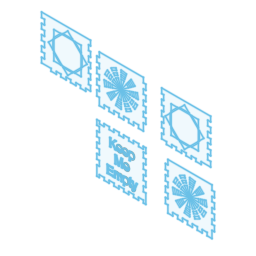
candelholder (Autodesk Fusion 360 design; units mm, degrees)
Autodesk Fusion 360 part; units mm, degrees
(part 1 of 3)
sketch "Sketch1" plane through (0, 0, 0) normal (0, 1, 0) x (1, 0, 0)
  line L0 (0, 0) -> (50, 0)
  line L1 (50, 0) -> (50, -50)
  line L2 (50, -50) -> (0, -50)
  line L3 (0, -50) -> (0, 0)
  line L4 (2.5, 0) -> (2.5, -2.5)
  line L5 (2.5, -2.5) -> (7.5, -2.5)
  line L6 (7.5, -2.5) -> (7.5, 0)
  line L7 (17.5, -2.5) -> (17.5, 0)
  line L8 (12.5, -2.5) -> (17.5, -2.5)
  line L9 (12.5, 0) -> (12.5, -2.5)
  line L10 (27.5, -2.5) -> (27.5, 0)
  line L11 (22.5, -2.5) -> (27.5, -2.5)
  line L12 (22.5, 0) -> (22.5, -2.5)
  line L13 (37.5, -2.5) -> (37.5, 0)
  line L14 (32.5, -2.5) -> (37.5, -2.5)
  line L15 (32.5, 0) -> (32.5, -2.5)
  line L16 (47.5, -2.5) -> (47.5, 0)
  line L17 (42.5, -2.5) -> (47.5, -2.5)
  line L18 (42.5, 0) -> (42.5, -2.5)
  line L19 (50, -25) -> (0, -25) construction
  line L20 (2.5, -50) -> (2.5, -47.5)
  line L21 (7.5, -47.5) -> (7.5, -50)
  line L22 (2.5, -47.5) -> (7.5, -47.5)
  line L23 (12.5, -50) -> (12.5, -47.5)
  line L24 (12.5, -47.5) -> (17.5, -47.5)
  line L25 (17.5, -47.5) -> (17.5, -50)
  line L26 (22.5, -50) -> (22.5, -47.5)
  line L27 (22.5, -47.5) -> (27.5, -47.5)
  line L28 (27.5, -47.5) -> (27.5, -50)
  line L29 (32.5, -50) -> (32.5, -47.5)
  line L30 (32.5, -47.5) -> (37.5, -47.5)
  line L31 (37.5, -47.5) -> (37.5, -50)
  line L32 (42.5, -50) -> (42.5, -47.5)
  line L33 (47.5, -47.5) -> (47.5, -50)
  line L34 (42.5, -47.5) -> (47.5, -47.5)
  line L35 (0, -5) -> (2.5, -5)
  line L36 (2.5, -5) -> (2.5, -10)
  line L37 (2.5, -10) -> (0, -10)
  line L38 (0, -15) -> (2.5, -15)
  line L39 (2.5, -15) -> (2.5, -20)
  line L40 (2.5, -20) -> (0, -20)
  line L41 (0, -25) -> (2.5, -25)
  line L42 (2.5, -25) -> (2.5, -30)
  line L43 (2.5, -30) -> (0, -30)
  line L44 (0, -35) -> (2.5, -35)
  line L45 (2.5, -35) -> (2.5, -40)
  line L46 (2.5, -40) -> (0, -40)
  line L47 (25, 0) -> (25, -50) construction
  line L48 (50, -5) -> (47.5, -5)
  line L49 (47.5, -10) -> (50, -10)
  line L50 (47.5, -5) -> (47.5, -10)
  line L51 (50, -15) -> (47.5, -15)
  line L52 (47.5, -15) -> (47.5, -20)
  line L53 (47.5, -20) -> (50, -20)
  line L54 (47.5, -25) -> (47.5, -30)
  line L55 (47.5, -30) -> (50, -30)
  line L56 (50, -25) -> (47.5, -25)
  line L57 (50, -35) -> (47.5, -35)
  line L58 (47.5, -35) -> (47.5, -40)
  line L59 (47.5, -40) -> (50, -40)
  dimension "d5" = 50
  dimension "d6" = 50
  dimension "d9" = 2.5
  dimension "d10" = 5
  dimension "d14" = 10
  dimension "d15" = 0
  dimension "d19" = 2.5
  dimension "d20" = 5
  dimension "d21" = 5
  dimension "d24" = -10
  dimension "d25" = 0
  constraint horizontal L0
  constraint vertical L1
  constraint horizontal L2
  constraint vertical L3
  constraint coincident L0.start L3.end
  constraint coincident L0 L4.start
  constraint perpendicular L0 L4
  constraint perpendicular L3 L5
  constraint coincident L0 L6.end
  constraint perpendicular L0 L6
  constraint midpoint L1 L19.start
  constraint midpoint L3 L19.end
  constraint symmetric L4.start L19 L20.start
  constraint symmetric L4.end L19 L20.end
  constraint symmetric L5.end L19 L21.start
  constraint symmetric L6.end L19 L21.end
  constraint symmetric L7.start L19 L24.end
  constraint symmetric L7.end L19 L25.end
  constraint symmetric L8.start L19 L23.end
  constraint symmetric L9.start L19 L23.start
  constraint symmetric L10.start L19 L27.end
  constraint symmetric L10.end L19 L28.end
  constraint symmetric L11.start L19 L26.end
  constraint symmetric L12.start L19 L26.start
  constraint symmetric L13.start L19 L30.end
  constraint symmetric L13.end L19 L31.end
  constraint symmetric L14.start L19 L29.end
  constraint symmetric L15.start L19 L29.start
  constraint symmetric L16.start L19 L33.start
  constraint symmetric L16.end L19 L33.end
  constraint symmetric L17.start L19 L32.end
  constraint symmetric L18.start L19 L32.start
  constraint coincident L3 L35.start
  constraint perpendicular L3 L35
  constraint perpendicular L19 L36
  constraint coincident L3 L37.end
  constraint perpendicular L3 L37
  constraint midpoint L0 L47.start
  constraint midpoint L2 L47.end
  constraint symmetric L35.start L47 L48.start
  constraint symmetric L35.end L47 L48.end
  constraint symmetric L36.end L47 L49.start
  constraint symmetric L37.end L47 L49.end
  constraint symmetric L38.start L47 L51.start
  constraint symmetric L38.end L47 L51.end
  constraint symmetric L39.end L47 L52.end
  constraint symmetric L40.end L47 L53.end
  constraint symmetric L19.end L47 L19.start
  constraint symmetric L41.end L47 L54.start
  constraint symmetric L42.end L47 L54.end
  constraint symmetric L43.end L47 L55.end
  constraint symmetric L44.start L47 L57.start
  constraint symmetric L44.end L47 L57.end
  constraint symmetric L45.end L47 L58.end
  constraint symmetric L46.end L47 L59.end
  measures "d5" distance of L0.start L0.end
  measures "d6" distance of L0.start L2.end
  measures "d9" distance of L4.start L4.end
  measures "d10" distance of L4.end L5.end
  measures "d19" distance of L35.start L35.end
  measures "d20" distance of L35.end L36.end
  measures "d21" distance of L0.start L35
extrude "Extrude1" add sketch "Sketch1" along normal blind 3 contours L0 L1 L2 L3 L4 L5 L6 L7 L8 L9 L10 L11 L12 L13 L14 L15 L16 L17 L18 L20 L21 L22 L23 L24 L25 L26 L27 L28 L29 L30 L31 L32 L33 L34 L35 L36 L37 L38 L39 L40 L41 L42 L43 L44 L45 L46 L48 L49 L50 L51 L52 L53 L54 L55 L56 L57 L58 L59 makes body 1
sketch "Sketch2" plane through (0, 0, 0) normal (1, 0, 0) x (0, 0, -1)
  line L0 (-46.9428, 61.6884) -> (3.0572, 61.6884)
  line L1 (3.0572, 61.6884) -> (3.0572, 11.6884)
  line L2 (3.0572, 11.6884) -> (-46.9428, 11.6884)
  line L3 (-46.9428, 11.6884) -> (-46.9428, 61.6884)
  line L4 (-7.7428, 61.6884) -> (-7.7428, 59.1884)
  line L5 (-7.7428, 59.1884) -> (-2.3428, 59.1884)
  line L6 (-2.3428, 59.1884) -> (-2.3428, 61.6884)
  line L7 (-12.3428, 59.1884) -> (-12.3428, 61.6884)
  line L8 (-17.7428, 59.1884) -> (-12.3428, 59.1884)
  line L9 (-17.7428, 61.6884) -> (-17.7428, 59.1884)
  line L10 (-22.3428, 59.1884) -> (-22.3428, 61.6884)
  line L11 (-27.7428, 59.1884) -> (-22.3428, 59.1884)
  line L12 (-27.7428, 61.6884) -> (-27.7428, 59.1884)
  line L13 (-32.3428, 59.1884) -> (-32.3428, 61.6884)
  line L14 (-37.7428, 59.1884) -> (-32.3428, 59.1884)
  line L15 (-37.7428, 61.6884) -> (-37.7428, 59.1884)
  line L16 (3.0572, 36.6884) -> (-46.9428, 36.6884) construction
  line L17 (-21.9428, 61.6884) -> (-21.9428, 11.6884) construction
  line L18 (-37.7428, 11.6884) -> (-37.7428, 14.1884)
  line L19 (-32.3428, 14.1884) -> (-32.3428, 11.6884)
  line L20 (-27.7428, 11.6884) -> (-27.7428, 14.1884)
  line L21 (-22.3428, 14.1884) -> (-22.3428, 11.6884)
  line L22 (-17.7428, 11.6884) -> (-17.7428, 14.1884)
  line L23 (-12.3428, 14.1884) -> (-12.3428, 11.6884)
  line L24 (-7.7428, 11.6884) -> (-7.7428, 14.1884)
  line L25 (-2.3428, 14.1884) -> (-2.3428, 11.6884)
  line L26 (3.0572, 59.1884) -> (0.5572, 59.1884)
  line L27 (0.5572, 54.1884) -> (3.0572, 54.1884)
  line L28 (3.0572, 49.1884) -> (0.5572, 49.1884)
  line L29 (0.5572, 44.1884) -> (3.0572, 44.1884)
  line L30 (3.0572, 39.1884) -> (0.5572, 39.1884)
  line L31 (0.5572, 36.6884) -> (0.5572, 34.1884)
  line L32 (0.5572, 34.1884) -> (3.0572, 34.1884)
  line L33 (3.0572, 29.1884) -> (0.5572, 29.1884)
  line L34 (0.5572, 24.1884) -> (3.0572, 24.1884)
  line L35 (3.0572, 19.1884) -> (0.5572, 19.1884)
  line L36 (0.5572, 14.1884) -> (3.0572, 14.1884)
  line L37 (-46.9428, 59.1884) -> (-44.4428, 59.1884)
  line L38 (-44.4428, 54.1884) -> (-46.9428, 54.1884)
  line L39 (-44.4428, 44.1884) -> (-46.9428, 44.1884)
  line L40 (-46.9428, 49.1884) -> (-44.4428, 49.1884)
  line L41 (-46.9428, 39.1884) -> (-44.4428, 39.1884)
  line L42 (-44.4428, 34.1884) -> (-46.9428, 34.1884)
  line L43 (-46.9428, 29.1884) -> (-44.4428, 29.1884)
  line L44 (-44.4428, 24.1884) -> (-46.9428, 24.1884)
  line L45 (-46.9428, 19.1884) -> (-44.4428, 19.1884)
  line L46 (-44.4428, 14.1884) -> (-46.9428, 14.1884)
  line L47 (-44.4428, 59.1884) -> (-37.7428, 59.1884)
  line L48 (-44.4428, 14.1884) -> (-37.7428, 14.1884)
  line L49 (0.5572, 14.1884) -> (-2.3428, 14.1884)
  line L50 (-2.3428, 59.1884) -> (0.5572, 59.1884)
  line L51 (-7.7428, 59.1884) -> (-32.3428, 59.1884)
  line L52 (0.5572, 49.1884) -> (0.5572, 54.1884)
  line L53 (-44.4428, 24.1884) -> (-44.4428, 19.1884)
  line L54 (-44.4428, 34.1884) -> (-44.4428, 29.1884)
  line L55 (-44.4428, 54.1884) -> (-44.4428, 49.1884)
  line L56 (-44.4428, 44.1884) -> (-44.4428, 39.1884)
  line L57 (-27.7428, 14.1884) -> (-32.3428, 14.1884)
  line L58 (-7.7428, 14.1884) -> (-12.3428, 14.1884)
  line L59 (-17.7428, 14.1884) -> (-22.3428, 14.1884)
  line L60 (0.5572, 19.1884) -> (0.5572, 24.1884)
  line L61 (0.5572, 29.1884) -> (0.5572, 36.6884)
  line L62 (0.5572, 39.1884) -> (0.5572, 44.1884)
  dimension "d29" = 50
  dimension "d30" = 50
  dimension "d31" = 2.5
  dimension "d32" = 5.4
  dimension "d33" = 5.4
  dimension "d36" = -10
  dimension "d37" = 0
  dimension "d38" = 2.5
  dimension "d39" = 5
  dimension "d40" = 2.5
  constraint horizontal L0
  constraint vertical L1
  constraint horizontal L2
  constraint vertical L3
  constraint coincident L0 L4.start
  constraint perpendicular L0 L4
  constraint perpendicular L4 L5
  constraint coincident L0 L6.end
  constraint perpendicular L0 L6
  constraint midpoint L1 L16.start
  constraint midpoint L3 L16.end
  constraint midpoint L0 L17.start
  constraint midpoint L2 L17.end
  constraint symmetric L4.start L16 L24.start
  constraint symmetric L4.end L16 L24.end
  constraint symmetric L5.end L16 L25.start
  constraint symmetric L6.end L16 L25.end
  constraint symmetric L7.start L16 L23.start
  constraint symmetric L7.end L16 L23.end
  constraint symmetric L8.start L16 L22.end
  constraint symmetric L9.start L16 L22.start
  constraint symmetric L10.start L16 L21.start
  constraint symmetric L10.end L16 L21.end
  constraint symmetric L11.start L16 L20.end
  constraint symmetric L12.start L16 L20.start
  constraint symmetric L13.start L16 L19.start
  constraint symmetric L13.end L16 L19.end
  constraint symmetric L14.start L16 L18.end
  constraint symmetric L15.start L16 L18.start
  constraint coincident L1 L26.start
  constraint perpendicular L1 L26
  constraint coincident L1 L27.end
  constraint perpendicular L1 L27
  constraint symmetric L17 L26.start L37.start
  constraint symmetric L17 L26.end L37.end
  constraint symmetric L17 L27.start L38.start
  constraint symmetric L17 L27.end L38.end
  constraint symmetric L17 L28.start L40.start
  constraint symmetric L17 L28.end L40.end
  constraint symmetric L17 L29.start L39.start
  constraint symmetric L17 L29.end L39.end
  constraint symmetric L17 L30.start L41.start
  constraint symmetric L17 L30.end L41.end
  constraint symmetric L17 L31.end L42.start
  constraint symmetric L17 L32.end L42.end
  constraint symmetric L17 L33.start L43.start
  constraint symmetric L17 L33.end L43.end
  constraint symmetric L17 L34.start L44.start
  constraint symmetric L17 L34.end L44.end
  constraint symmetric L17 L35.start L45.start
  constraint symmetric L17 L35.end L45.end
  constraint symmetric L17 L36.start L46.start
  constraint symmetric L17 L36.end L46.end
  constraint collinear L53 L55
  constraint collinear L54 L55
  constraint collinear L55 L56
  constraint collinear L57 L58
  constraint collinear L58 L59
  constraint collinear L60 L61
  constraint coincident L16 L31.start
  constraint collinear L61 L62
  measures "d29" distance of L0.start L0.end
  measures "d30" distance of L0.start L2.end
  measures "d31" distance of L4.start L4.end
  measures "d32" distance of L4.end L5.end
  measures "d33" horizontal distance of L0.end L5.end
  measures "d38" distance of L26.start L26.end
  measures "d39" distance of L26.end L27.start
  measures "d40" distance of L0 L26
extrude "Extrude2" add sketch "Sketch2" along normal blind 3 separate body contours L1 L2 L3 L5 L8 L11 L14 L18 L19 L20 L21 L22 L23 L24 L25 L26 L27 L28 L29 L30 L32 L33 L34 L35 L36 L37 L38 L39 L40 L41 L42 L43 L44 L45 L46 L47 L48 L49 L50 L51 L52 L53 L54 L55 L56 L57 L58 L59 L60 L61 L62 makes body 2
copy_body "Body->Comp1" bodies 1 removing the originals makes body 3 in component "Component"
copy_body "Body->Comp3" bodies 2 removing the originals makes body 4 in component "Component''"
extrude "Extrude1'" cut 5 faces at (1, 27.5218, -3.0572) (1, 17.5218, -3.0572) (1, 37.5218, -3.0572) (1, 47.5218, -3.0572) (1, 57.5218, -3.0572) along direction (0, 0, 1) blind 0.5 on bodies 4 bodies 4 in component "Component''"
extrude "Extrude2'" add 5 faces at (1, 25.8551, 46.9428) (1, 15.8551, 46.9428) (1, 35.8551, 46.9428) (1, 45.8551, 46.9428) (1, 55.8551, 46.9428) along direction (0, 0, 1) blind 0.5 on bodies 4 bodies 4 in component "Component''"
sketch "Sketch3" plane through (0, 0, 0) normal (0, 0, 1) x (1, 0, 0)
  line L0 (0, 0) -> (50, 0)
  line L1 (50, 0) -> (50, 47.5)
  line L2 (50, 47.5) -> (0, 47.5)
  line L3 (0, 47.5) -> (0, 0)
  line L4 (47.5, 37.5) -> (47.5, 42.5)
  line L5 (47.5, 42.5) -> (50.5, 42.5)
  line L6 (50.5, 42.5) -> (50.5, 37.5)
  line L7 (50.5, 37.5) -> (47.5, 37.5)
  line L8 (47.5, 27.5) -> (47.5, 32.5)
  line L9 (47.5, 32.5) -> (50.5, 32.5)
  line L10 (50.5, 32.5) -> (50.5, 27.5)
  line L11 (50.5, 27.5) -> (47.5, 27.5)
  line L12 (47.5, 17.5) -> (47.5, 22.5)
  line L13 (47.5, 22.5) -> (50.5, 22.5)
  line L14 (50.5, 22.5) -> (50.5, 17.5)
  line L15 (50.5, 17.5) -> (47.5, 17.5)
  line L16 (47.5, 7.5) -> (47.5, 12.5)
  line L17 (47.5, 12.5) -> (50.5, 12.5)
  line L18 (50.5, 12.5) -> (50.5, 7.5)
  line L19 (50.5, 7.5) -> (47.5, 7.5)
  line L20 (47.5, 0) -> (42.5, 0)
  line L21 (42.5, 0) -> (42.5, 3)
  line L22 (42.5, 3) -> (47.5, 3)
  line L23 (47.5, 3) -> (47.5, 0)
  line L24 (37.5, 0) -> (32.5, 0)
  line L25 (32.5, 0) -> (32.5, 3)
  line L26 (32.5, 3) -> (37.5, 3)
  line L27 (37.5, 3) -> (37.5, 0)
  line L28 (27.5, 0) -> (22.5, 0)
  line L29 (22.5, 0) -> (22.5, 3)
  line L30 (22.5, 3) -> (27.5, 3)
  line L31 (27.5, 3) -> (27.5, 0)
  line L32 (17.5, 0) -> (12.5, 0)
  line L33 (12.5, 0) -> (12.5, 3)
  line L34 (12.5, 3) -> (17.5, 3)
  line L35 (17.5, 3) -> (17.5, 0)
  line L36 (7.5, 0) -> (2.5, 0)
  line L37 (2.5, 0) -> (2.5, 3)
  line L38 (2.5, 3) -> (7.5, 3)
  line L39 (7.5, 3) -> (7.5, 0)
  line L40 (-0.5, 7.5) -> (-0.5, 12.5)
  line L41 (-0.5, 12.5) -> (2.5, 12.5)
  line L42 (2.5, 12.5) -> (2.5, 7.5)
  line L43 (2.5, 7.5) -> (-0.5, 7.5)
  line L44 (-0.5, 17.5) -> (-0.5, 22.5)
  line L45 (-0.5, 22.5) -> (2.5, 22.5)
  line L46 (2.5, 22.5) -> (2.5, 17.5)
  line L47 (2.5, 17.5) -> (-0.5, 17.5)
  line L48 (-0.5, 27.5) -> (-0.5, 32.5)
  line L49 (-0.5, 32.5) -> (2.5, 32.5)
  line L50 (2.5, 32.5) -> (2.5, 27.5)
  line L51 (2.5, 27.5) -> (-0.5, 27.5)
  line L52 (-0.5, 37.5) -> (-0.5, 42.5)
  line L53 (-0.5, 42.5) -> (2.5, 42.5)
  line L54 (2.5, 42.5) -> (2.5, 37.5)
  line L55 (2.5, 37.5) -> (-0.5, 37.5)
  line L56 (2.5, 42.5) -> (2.5, 47.5)
  line L57 (2.5, 32.5) -> (2.5, 37.5)
  line L58 (2.5, 22.5) -> (2.5, 27.5)
  line L59 (2.5, 12.5) -> (2.5, 17.5)
  line L60 (2.5, 2.5) -> (2.5, 7.5)
  line L61 (47.5, 42.5) -> (50.5, 42.5)
  line L62 (50.5, 32.5) -> (50.5, 37.5)
  line L63 (50.5, 37.5) -> (50.5, 42.5)
  line L64 (50.5, 42.5) -> (50.5, 47.5)
  line L65 (50.5, 47.5) -> (50.5, 42.5)
  line L66 (50.5, 42.5) -> (50.5, 37.5)
  line L67 (50.5, 37.5) -> (50.5, 32.5)
  line L68 (50.5, 32.5) -> (50.5, 27.5)
  line L69 (50.5, 27.5) -> (50.5, 22.5)
  line L70 (50.5, 22.5) -> (50.5, 17.5)
  line L71 (50.5, 17.5) -> (50.5, 12.5)
  line L72 (50.5, 12.5) -> (50.5, 7.5)
  line L73 (50.5, 7.5) -> (50.5, 2.5)
  line L74 (50.5, 2.5) -> (50.5, 0)
  line L75 (50.5, 0) -> (50.5, 2.5)
  line L76 (50.5, 2.5) -> (50.5, 0)
  line L77 (50.5, 0) -> (50.5, 2.5)
  line L78 (50.5, 2.5) -> (50.5, 0)
  line L79 (50.5, 0) -> (50.5, 2.5)
  line L80 (50.5, 2.5) -> (50.5, 0)
  line L81 (50.5, 0) -> (50.5, 2.5)
  line L82 (50.5, 2.5) -> (50.5, 7.5)
  line L83 (50.5, 7.5) -> (50.5, 12.5)
  line L84 (50.5, 12.5) -> (50.5, 17.5)
  line L85 (50.5, 17.5) -> (50.5, 22.5)
  line L86 (50.5, 22.5) -> (50.5, 27.5)
  line L87 (50.5, 27.5) -> (50.5, 32.5)
  line L88 (-0.5, 37.5) -> (-0.5, 32.5)
  line L89 (-0.5, 32.5) -> (-0.5, 27.5)
  line L90 (-0.5, 27.5) -> (-0.5, 22.5)
  line L91 (-0.5, 22.5) -> (-0.5, 17.5)
  line L92 (-0.5, 17.5) -> (-0.5, 12.5)
  line L93 (-0.5, 12.5) -> (-0.5, 7.5)
  line L94 (-0.5, 7.5) -> (-0.5, 2.5)
  line L95 (-0.5, 2.5) -> (-0.5, 0)
  line L96 (-0.5, 0) -> (-0.5, 2.5)
  line L97 (-0.5, 2.5) -> (-0.5, 0)
  line L98 (-0.5, 0) -> (-0.5, 2.5)
  line L99 (-0.5, 2.5) -> (-0.5, 0)
  line L100 (-0.5, 0) -> (-0.5, 2.5)
  line L101 (-0.5, 2.5) -> (-0.5, 0)
  line L102 (-0.5, 0) -> (-0.5, 2.5)
  line L103 (-0.5, 2.5) -> (-0.5, 7.5)
  line L104 (-0.5, 7.5) -> (-0.5, 12.5)
  line L105 (-0.5, 12.5) -> (-0.5, 17.5)
  line L106 (-0.5, 17.5) -> (-0.5, 22.5)
  line L107 (-0.5, 22.5) -> (-0.5, 27.5)
  line L108 (-0.5, 27.5) -> (-0.5, 32.5)
  line L109 (-0.5, 32.5) -> (-0.5, 37.5)
  line L110 (-0.5, 37.5) -> (-0.5, 42.5)
  line L111 (-0.5, 42.5) -> (-0.5, 47.5)
  line L112 (-0.5, 47.5) -> (-0.5, 42.5)
  line L113 (-0.5, 42.5) -> (-0.5, 37.5)
  line L114 (2.5, 0) -> (0, 0)
  line L115 (0, 0) -> (2.5, 0)
  line L116 (2.5, 0) -> (7.5, 0)
  line L117 (7.5, 0) -> (12.5, 0)
  line L118 (12.5, 0) -> (17.5, 0)
  line L119 (17.5, 0) -> (22.5, 0)
  line L120 (22.5, 0) -> (27.5, 0)
  line L121 (27.5, 0) -> (32.5, 0)
  line L122 (32.5, 0) -> (37.5, 0)
  line L123 (37.5, 0) -> (42.5, 0)
  line L124 (42.5, 0) -> (47.5, 0)
  line L125 (47.5, 0) -> (50, 0)
  line L126 (50, 0) -> (47.5, 0)
  line L127 (47.5, 0) -> (50, 0)
  line L128 (50, 0) -> (47.5, 0)
  line L129 (47.5, 0) -> (50, 0)
  line L130 (50, 0) -> (47.5, 0)
  line L131 (47.5, 0) -> (50, 0)
  line L132 (50, 0) -> (47.5, 0)
  line L133 (47.5, 0) -> (50, 0)
  line L134 (50, 0) -> (47.5, 0)
  line L135 (47.5, 0) -> (42.5, 0)
  line L136 (42.5, 0) -> (37.5, 0)
  line L137 (37.5, 0) -> (32.5, 0)
  line L138 (32.5, 0) -> (27.5, 0)
  line L139 (27.5, 0) -> (22.5, 0)
  line L140 (22.5, 0) -> (17.5, 0)
  line L141 (17.5, 0) -> (12.5, 0)
  line L142 (12.5, 0) -> (7.5, 0)
  line L143 (7.5, 0) -> (2.5, 0)
  line L144 (2.5, 0) -> (0, 0)
  line L145 (0, 0) -> (2.5, 0)
  line L146 (2.5, 0) -> (0, 0)
  line L147 (0, 0) -> (2.5, 0)
  line L148 (2.5, 0) -> (0, 0)
  line L149 (0, 0) -> (2.5, 0)
  line L150 (2.5, 0) -> (0, 0)
  line L151 (0, 0) -> (2.5, 0)
  line L152 (47.5, 37.5) -> (47.5, 32.5)
  line L153 (47.5, 32.5) -> (47.5, 27.5)
  line L154 (47.5, 27.5) -> (47.5, 22.5)
  line L155 (47.5, 22.5) -> (47.5, 17.5)
  line L156 (47.5, 17.5) -> (47.5, 12.5)
  line L157 (47.5, 12.5) -> (47.5, 7.5)
  line L158 (47.5, 7.5) -> (47.5, 2.5)
  line L159 (47.5, 2.5) -> (47.5, 0)
  line L160 (47.5, 0) -> (47.5, 2.5)
  line L161 (47.5, 2.5) -> (47.5, 0)
  line L162 (47.5, 0) -> (47.5, 2.5)
  line L163 (47.5, 2.5) -> (47.5, 0)
  line L164 (47.5, 0) -> (47.5, 2.5)
  line L165 (47.5, 2.5) -> (47.5, 0)
  line L166 (47.5, 0) -> (47.5, 2.5)
  line L167 (47.5, 2.5) -> (47.5, 7.5)
  line L168 (47.5, 7.5) -> (47.5, 12.5)
  line L169 (47.5, 12.5) -> (47.5, 17.5)
  line L170 (47.5, 17.5) -> (47.5, 22.5)
  line L171 (47.5, 22.5) -> (47.5, 27.5)
  line L172 (47.5, 27.5) -> (47.5, 32.5)
  line L173 (47.5, 32.5) -> (47.5, 37.5)
  line L174 (47.5, 37.5) -> (47.5, 42.5)
  line L175 (47.5, 42.5) -> (47.5, 47.5)
  line L176 (47.5, 47.5) -> (47.5, 42.5)
  line L177 (47.5, 42.5) -> (47.5, 37.5)
  line L178 (0, 3) -> (2.5, 3)
  line L179 (2.5, 3) -> (0, 3)
  line L180 (0, 3) -> (2.5, 3)
  line L181 (2.5, 3) -> (0, 3)
  line L182 (0, 3) -> (2.5, 3)
  line L183 (2.5, 3) -> (0, 3)
  line L184 (0, 3) -> (2.5, 3)
  line L185 (2.5, 3) -> (0, 3)
  line L186 (0, 3) -> (2.5, 3)
  line L187 (2.5, 3) -> (7.5, 3)
  line L188 (7.5, 3) -> (12.5, 3)
  line L189 (12.5, 3) -> (17.5, 3)
  line L190 (17.5, 3) -> (22.5, 3)
  line L191 (22.5, 3) -> (27.5, 3)
  line L192 (27.5, 3) -> (32.5, 3)
  line L193 (32.5, 3) -> (37.5, 3)
  line L194 (37.5, 3) -> (42.5, 3)
  line L195 (42.5, 3) -> (47.5, 3)
  line L196 (47.5, 3) -> (50, 3)
  line L197 (50, 3) -> (47.5, 3)
  line L198 (47.5, 3) -> (50, 3)
  line L199 (50, 3) -> (47.5, 3)
  line L200 (47.5, 3) -> (50, 3)
  line L201 (50, 3) -> (47.5, 3)
  line L202 (47.5, 3) -> (50, 3)
  line L203 (50, 3) -> (47.5, 3)
  line L204 (47.5, 3) -> (50, 3)
  line L205 (50, 3) -> (47.5, 3)
  line L206 (47.5, 3) -> (42.5, 3)
  line L207 (42.5, 3) -> (37.5, 3)
  line L208 (37.5, 3) -> (32.5, 3)
  line L209 (32.5, 3) -> (27.5, 3)
  line L210 (27.5, 3) -> (22.5, 3)
  line L211 (22.5, 3) -> (17.5, 3)
  line L212 (17.5, 3) -> (12.5, 3)
  line L213 (12.5, 3) -> (7.5, 3)
  line L214 (7.5, 3) -> (2.5, 3)
  line L215 (2.5, 3) -> (0, 3)
  dimension "d71" = 47.5
  dimension "d72" = 50
  constraint horizontal L0
  constraint vertical L1
  constraint horizontal L2
  constraint vertical L3
  constraint coincident L0.start L3.end
  measures "d71" distance of L0.start L2.end
  measures "d72" distance of L1.end L2.end
sketch "Sketch4" plane through (25, 25.25, -65) normal (0, 0, 1) x (1, 0, 0)
extrude "Extrude3" add sketch "Sketch3" against normal blind 3 separate body contours L0 L36 L37 L38 L39 L60 L116 L143 L187 L214 | L3 L41 L42 L43 | L2 L4 L8 L12 L16 L22 L26 L30 L34 L38 L42 L46 L50 L54 L56 L57 L58 L59 L60 L152 L153 L154 L155 L156 L157 L158 L167 L168 L169 L170 L171 L172 L173 L174 L175 L176 L177 L187 L188 L189 L190 L191 L192 L193 L194 L195 L206 L207 L208 L209 L210 L211 L212 L213 L214 | L0 L32 L33 L34 L35 L118 L141 L189 L212 | L3 L45 L46 L47 | L0 L28 L29 L30 L31 L120 L139 L191 L210 | L3 L49 L50 L51 | L0 L24 L25 L26 L27 L122 L137 L193 L208 | L3 L53 L54 L55 | L0 L20 L21 L22 L23 L124 L135 L158 L159 L160 L161 L162 L163 L164 L165 L166 L167 L195 L206 | L1 L16 L17 L19 L157 L168 | L1 L4 L5 L7 L61 L174 L177 | L1 L12 L13 L15 L155 L170 | L1 L8 L9 L11 L153 L172 makes body 5
extrude "Extrude4" add 1 faces at (0.8333, 42.5, -1) along direction (0, 1, 0) blind 0.2 on bodies 5 bodies 5
extrude "Extrude5" add 1 faces at (1.6667, 37.5, -1) along direction (0, -1, 0) blind 0.2 on bodies 5 bodies 5
extrude "Extrude6" add 1 faces at (1.6667, 27.5, -1) along direction (0, -1, 0) blind 0.2 on bodies 5 bodies 5
extrude "Extrude7" add 1 faces at (1.6667, 17.5, -1) along direction (0, -1, 0) blind 0.2 on bodies 5 bodies 5
extrude "Extrude8" add 1 faces at (1.6667, 7.5, -1) along direction (0, -1, 0) blind 0.2 on bodies 5 bodies 5
extrude "Extrude9" add 1 faces at (0.8333, 32.5, -1) along direction (0, 1, 0) blind 0.2 on bodies 5 bodies 5
extrude "Extrude10" add 1 faces at (0.8333, 22.5, -1) along direction (0, 1, 0) blind 0.2 on bodies 5 bodies 5
extrude "Extrude11" add 1 faces at (0.8333, 12.5, -1) along direction (0, 1, 0) blind 0.2 on bodies 5 bodies 5
extrude "Extrude1''" add 1 faces at (7.5, 1, 1.6667) along direction (-1, 0, 0) blind 0.2 on bodies 3 bodies 3 in component "Component"
extrude "Extrude2''" add 1 faces at (17.5, 1, 1.6667) along direction (-1, 0, 0) blind 0.2 on bodies 3 bodies 3 in component "Component"
extrude "Extrude3'" add 1 faces at (27.5, 1, 1.6667) along direction (-1, 0, 0) blind 0.2 on bodies 3 bodies 3 in component "Component"
extrude "Extrude4'" add 1 faces at (37.5, 1, 1.6667) along direction (-1, 0, 0) blind 0.2 on bodies 3 bodies 3 in component "Component"
extrude "Extrude5'" add 1 faces at (47.5, 1, 1.6667) along direction (-1, 0, 0) blind 0.2 on bodies 3 bodies 3 in component "Component"
extrude "Extrude6'" add 1 faces at (42.5, 1, 0.8333) along direction (1, 0, 0) blind 0.2 on bodies 3 bodies 3 in component "Component"
extrude "Extrude7'" add 1 faces at (32.5, 1, 0.8333) along direction (1, 0, 0) blind 0.2 on bodies 3 bodies 3 in component "Component"
extrude "Extrude8'" add 1 faces at (22.5, 1, 0.8333) along direction (1, 0, 0) blind 0.2 on bodies 3 bodies 3 in component "Component"
extrude "Extrude9'" add 1 faces at (12.5, 1, 0.8333) along direction (1, 0, 0) blind 0.2 on bodies 3 bodies 3 in component "Component"
extrude "Extrude10'" add 1 faces at (2.5, 1, 0.8333) along direction (1, 0, 0) blind 0.2 on bodies 3 bodies 3 in component "Component"
extrude "Extrude12" add 1 faces at (49.1667, 7.5, -1) along direction (0, -1, 0) blind 0.2 on bodies 5 bodies 5
extrude "Extrude13" add 1 faces at (49.1667, 17.5, -1) along direction (0, -1, 0) blind 0.2 on bodies 5 bodies 5
extrude "Extrude14" add 1 faces at (49.1667, 27.5, -1) along direction (0, -1, 0) blind 0.2 on bodies 5 bodies 5
extrude "Extrude15" add 1 faces at (49.1667, 37.5, -1) along direction (0, -1, 0) blind 0.2 on bodies 5 bodies 5
extrude "Extrude16" add 1 faces at (48.3333, 42.5, -1) along direction (0, 1, 0) blind 0.2 on bodies 5 bodies 5
extrude "Extrude17" add 1 faces at (48.3333, 32.5, -1) along direction (0, 1, 0) blind 0.2 on bodies 5 bodies 5
extrude "Extrude18" add 1 faces at (48.3333, 22.5, -1) along direction (0, 1, 0) blind 0.2 on bodies 5 bodies 5
extrude "Extrude19" add 1 faces at (48.3333, 12.5, -1) along direction (0, 1, 0) blind 0.2 on bodies 5 bodies 5
copy_body "Body->Comp4" bodies 5 removing the originals makes body 6 in component "Component'''"
sketch "Sketch9" plane through (0, 0, 26.4903) normal (0, 0, 1) x (1, 0, 0)
  line L0 (0, 41.4903) -> (2.5, 41.4903)
  line L1 (2.5, 41.4903) -> (2.5, 36.4903)
  line L2 (2.5, 36.4903) -> (0, 36.4903)
  line L3 (0, 36.4903) -> (0, 31.4903)
  line L4 (0, 31.4903) -> (2.5, 31.4903)
  line L5 (2.5, 31.4903) -> (2.5, 26.4903)
  line L6 (2.5, 26.4903) -> (0, 26.4903)
  line L7 (0, 26.4903) -> (0, 21.4903)
  line L8 (0, 21.4903) -> (2.5, 21.4903)
  line L9 (2.5, 21.4903) -> (2.5, 16.4903)
  line L10 (2.5, 16.4903) -> (0, 16.4903)
  line L11 (0, 16.4903) -> (0, 11.4903)
  line L12 (0, 11.4903) -> (2.5, 11.4903)
  line L13 (2.5, 11.4903) -> (2.5, 6.4903)
  line L14 (2.5, 6.4903) -> (0, 6.4903)
  line L15 (0, 6.4903) -> (0, -3.5097)
  line L16 (0, -3.5097) -> (2.5, -3.5097)
  line L17 (2.5, -3.5097) -> (2.5, -1.0097)
  line L18 (2.5, -1.0097) -> (7.5, -1.0097)
  line L19 (7.5, -1.0097) -> (7.5, -3.5097)
  line L20 (7.5, -3.5097) -> (12.5, -3.5097)
  line L21 (12.5, -3.5097) -> (12.5, -1.0097)
  line L22 (12.5, -1.0097) -> (17.5, -1.0097)
  line L23 (17.5, -1.0097) -> (17.5, -3.5097)
  line L24 (17.5, -3.5097) -> (22.5, -3.5097)
  line L25 (22.5, -3.5097) -> (22.5, -1.0097)
  line L26 (22.5, -1.0097) -> (27.5, -1.0097)
  line L27 (27.5, -1.0097) -> (27.5, -3.5097)
  line L28 (27.5, -3.5097) -> (32.5, -3.5097)
  line L29 (32.5, -3.5097) -> (32.5, -1.0097)
  line L30 (32.5, -1.0097) -> (37.5, -1.0097)
  line L31 (37.5, -1.0097) -> (37.5, -3.5097)
  line L32 (37.5, -3.5097) -> (42.5, -3.5097)
  line L33 (42.5, -3.5097) -> (42.5, -1.0097)
  line L34 (42.5, -1.0097) -> (47.5, -1.0097)
  line L35 (47.5, -1.0097) -> (47.5, -3.5097)
  line L36 (47.5, -3.5097) -> (50, -3.5097)
  line L37 (50, -3.5097) -> (50, 6.4903)
  line L38 (50, 6.4903) -> (47.5, 6.4903)
  line L39 (47.5, 6.4903) -> (47.5, 11.4903)
  line L40 (47.5, 11.4903) -> (50, 11.4903)
  line L41 (50, 11.4903) -> (50, 16.4903)
  line L42 (50, 16.4903) -> (47.5, 16.4903)
  line L43 (47.5, 16.4903) -> (47.5, 21.4903)
  line L44 (47.5, 21.4903) -> (50, 21.4903)
  line L45 (50, 21.4903) -> (50, 26.4903)
  line L46 (50, 26.4903) -> (47.5, 26.4903)
  line L47 (47.5, 26.4903) -> (47.5, 31.4903)
  line L48 (47.5, 31.4903) -> (50, 31.4903)
  line L49 (50, 31.4903) -> (50, 36.4903)
  line L50 (50, 36.4903) -> (47.5, 36.4903)
  line L51 (47.5, 36.4903) -> (47.5, 41.4903)
  line L52 (47.5, 41.4903) -> (50, 41.4903)
  line L53 (50, 41.4903) -> (50, 46.4903)
  line L54 (50, 46.4903) -> (47.3, 46.4903)
  line L55 (47.3, 46.4903) -> (47.3, 43.9903)
  line L56 (47.3, 43.9903) -> (42.7, 43.9903)
  line L57 (42.7, 43.9903) -> (42.7, 46.4903)
  line L58 (42.7, 46.4903) -> (37.3, 46.4903)
  line L59 (37.3, 46.4903) -> (37.3, 43.9903)
  line L60 (37.3, 43.9903) -> (32.7, 43.9903)
  line L61 (32.7, 43.9903) -> (32.7, 46.4903)
  line L62 (32.7, 46.4903) -> (27.3, 46.4903)
  line L63 (27.3, 46.4903) -> (27.3, 43.9903)
  line L64 (27.3, 43.9903) -> (22.7, 43.9903)
  line L65 (22.7, 43.9903) -> (22.7, 46.4903)
  line L66 (22.7, 46.4903) -> (17.3, 46.4903)
  line L67 (17.3, 46.4903) -> (17.3, 43.9903)
  line L68 (17.3, 43.9903) -> (12.7, 43.9903)
  line L69 (12.7, 43.9903) -> (12.7, 46.4903)
  line L70 (12.7, 46.4903) -> (7.3, 46.4903)
  line L71 (7.3, 46.4903) -> (7.3, 43.9903)
  line L72 (7.3, 43.9903) -> (2.7, 43.9903)
  line L73 (2.7, 43.9903) -> (2.7, 46.4903)
  line L74 (2.7, 46.4903) -> (0, 46.4903)
  line L75 (0, 46.4903) -> (0, 41.4903)
  line L76 (13.2269, 29.2859) -> (13.2269, 37.2859)
  line L77 (13.2269, 37.2859) -> (14.2855, 37.2859)
  line L78 (14.2855, 37.2859) -> (14.2855, 33.3186)
  line L79 (14.2855, 33.3186) -> (18.2583, 37.2859)
  line L80 (18.2583, 37.2859) -> (19.6935, 37.2859)
  line L81 (19.6935, 37.2859) -> (16.3374, 34.0444)
  line L82 (16.3374, 34.0444) -> (19.8408, 29.2859)
  line L83 (19.8408, 29.2859) -> (18.4438, 29.2859)
  line L84 (18.4438, 29.2859) -> (15.5952, 33.335)
  line L85 (15.5952, 33.335) -> (14.2855, 32.0581)
  line L86 (14.2855, 32.0581) -> (14.2855, 29.2859)
  line L87 (14.2855, 29.2859) -> (13.2269, 29.2859)
  line L88 (24.5666, 31.1522) -> (25.5816, 31.0267)
  spline S0 degree 3 poles (25.5816, 31.0267) (25.4883, 30.7497) (25.3079, 30.2138) (24.8927, 29.831) (24.6921, 29.646) knots 0 0 0 0 0.086093 0.166606 0.166606 0.166606 0.166606
  spline S1 degree 3 poles (24.6921, 29.646) (24.4518, 29.5029) (23.9418, 29.1991) (23.3475, 29.1702) (23.0332, 29.1549) knots 0 0 0 0 0.08261 0.175377 0.175377 0.175377 0.175377
  spline S2 degree 3 poles (23.0332, 29.1549) (22.6376, 29.1811) (21.8812, 29.2313) (21.296, 29.7097) (21.0168, 29.938) knots 0 0 0 0 0.115653 0.221163 0.221163 0.221163 0.221163
  spline S3 degree 3 poles (21.0168, 29.938) (20.7998, 30.2406) (20.3312, 30.8944) (20.2926, 31.7011) (20.2719, 32.1345) knots 0 0 0 0 0.109405 0.236358 0.236358 0.236358 0.236358
  spline S4 degree 3 poles (20.2719, 32.1345) (20.2923, 32.5821) (20.3302, 33.4131) (20.8057, 34.0916) (21.025, 34.4046) knots 0 0 0 0 0.131235 0.243597 0.243597 0.243597 0.243597
  spline S5 degree 3 poles (21.025, 34.4046) (21.2992, 34.6401) (21.8609, 35.1226) (22.6002, 35.1819) (22.9786, 35.2122) knots 0 0 0 0 0.105595 0.216319 0.216319 0.216319 0.216319
  spline S6 degree 3 poles (22.9786, 35.2122) (23.3457, 35.182) (24.065, 35.1229) (24.6105, 34.6517) (24.8776, 34.4209) knots 0 0 0 0 0.10743 0.210533 0.210533 0.210533 0.210533
  spline S7 degree 3 poles (24.8776, 34.4209) (25.0922, 34.1141) (25.5575, 33.4484) (25.5944, 32.6336) (25.6143, 32.1945) knots 0 0 0 0 0.110094 0.238839 0.238839 0.238839 0.238839
  spline S8 degree 3 poles (25.6143, 32.1945) (25.614, 32.1581) (25.6131, 32.0708) (25.6104, 31.9835) (25.6089, 31.9325) knots 0 0 0 0 0.010915 0.0262 0.0262 0.0262 0.0262
  line L89 (25.6089, 31.9325) -> (21.2869, 31.9325)
  spline S9 degree 3 poles (21.2869, 31.9325) (21.3153, 31.6416) (21.3677, 31.1047) (21.6828, 30.6694) (21.8271, 30.4701) knots 0 0 0 0 0.08586 0.158415 0.158415 0.158415 0.158415
  spline S10 degree 3 poles (21.8271, 30.4701) (22.0001, 30.322) (22.3494, 30.0232) (22.8074, 29.9829) (23.0386, 29.9626) knots 0 0 0 0 0.066533 0.134307 0.134307 0.134307 0.134307
  spline S11 degree 3 poles (23.0386, 29.9626) (23.2097, 29.9727) (23.5407, 29.9922) (23.824, 30.1636) (23.9608, 30.2463) knots 0 0 0 0 0.050568 0.097791 0.097791 0.097791 0.097791
  spline S12 degree 3 poles (23.9608, 30.2463) (24.0842, 30.3628) (24.3544, 30.6178) (24.4919, 30.964) (24.5666, 31.1522) knots 0 0 0 0 0.050293 0.110147 0.110147 0.110147 0.110147
  line L90 (21.3415, 32.7402) -> (24.5775, 32.7402)
  spline S13 degree 3 poles (24.5775, 32.7402) (24.5526, 32.9595) (24.508, 33.3534) (24.299, 33.6885) (24.2064, 33.837) knots 0 0 0 0 0.065203 0.117085 0.117085 0.117085 0.117085
  spline S14 degree 3 poles (24.2064, 33.837) (24.0378, 34.0026) (23.6992, 34.3351) (23.2268, 34.3813) (22.9895, 34.4046) knots 0 0 0 0 0.068671 0.137943 0.137943 0.137943 0.137943
  spline S15 degree 3 poles (22.9895, 34.4046) (22.7739, 34.3867) (22.3483, 34.3514) (22.0158, 34.0837) (21.8517, 33.9516) knots 0 0 0 0 0.063299 0.124994 0.124994 0.124994 0.124994
  spline S16 degree 3 poles (21.8517, 33.9516) (21.7149, 33.7827) (21.4285, 33.4291) (21.3713, 32.9765) (21.3415, 32.7402) knots 0 0 0 0 0.063909 0.133798 0.133798 0.133798 0.133798
  line L91 (30.7821, 31.1522) -> (31.7971, 31.0267)
  spline S17 degree 3 poles (31.7971, 31.0267) (31.7039, 30.7497) (31.5234, 30.2138) (31.1083, 29.831) (30.9076, 29.646) knots 0 0 0 0 0.086093 0.166606 0.166606 0.166606 0.166606
  spline S18 degree 3 poles (30.9076, 29.646) (30.6674, 29.5029) (30.1574, 29.1991) (29.5631, 29.1702) (29.2487, 29.1549) knots 0 0 0 0 0.082609 0.175376 0.175376 0.175376 0.175376
  spline S19 degree 3 poles (29.2487, 29.1549) (28.8532, 29.1811) (28.0967, 29.2313) (27.5115, 29.7097) (27.2323, 29.938) knots 0 0 0 0 0.115653 0.221163 0.221163 0.221163 0.221163
  spline S20 degree 3 poles (27.2323, 29.938) (27.0154, 30.2406) (26.5467, 30.8944) (26.5082, 31.7011) (26.4874, 32.1345) knots 0 0 0 0 0.109405 0.236358 0.236358 0.236358 0.236358
  spline S21 degree 3 poles (26.4874, 32.1345) (26.5079, 32.5821) (26.5458, 33.4131) (27.0212, 34.0916) (27.2405, 34.4046) knots 0 0 0 0 0.131235 0.243597 0.243597 0.243597 0.243597
  spline S22 degree 3 poles (27.2405, 34.4046) (27.5147, 34.6401) (28.0765, 35.1226) (28.8157, 35.1819) (29.1941, 35.2122) knots 0 0 0 0 0.105595 0.216319 0.216319 0.216319 0.216319
  spline S23 degree 3 poles (29.1941, 35.2122) (29.5612, 35.182) (30.2806, 35.1229) (30.826, 34.6517) (31.0932, 34.4209) knots 0 0 0 0 0.10743 0.210533 0.210533 0.210533 0.210533
  spline S24 degree 3 poles (31.0932, 34.4209) (31.3077, 34.1141) (31.7731, 33.4484) (31.81, 32.6336) (31.8299, 32.1945) knots 0 0 0 0 0.110094 0.238839 0.238839 0.238839 0.238839
  spline S25 degree 3 poles (31.8299, 32.1945) (31.8295, 32.1581) (31.8287, 32.0708) (31.826, 31.9835) (31.8244, 31.9325) knots 0 0 0 0 0.010915 0.0262 0.0262 0.0262 0.0262
  line L92 (31.8244, 31.9325) -> (27.5025, 31.9325)
  spline S26 degree 3 poles (27.5025, 31.9325) (27.5308, 31.6416) (27.5832, 31.1047) (27.8984, 30.6694) (28.0427, 30.4701) knots 0 0 0 0 0.08586 0.158415 0.158415 0.158415 0.158415
  spline S27 degree 3 poles (28.0427, 30.4701) (28.2157, 30.322) (28.5649, 30.0232) (29.023, 29.9829) (29.2542, 29.9626) knots 0 0 0 0 0.066533 0.134307 0.134307 0.134307 0.134307
  spline S28 degree 3 poles (29.2542, 29.9626) (29.4253, 29.9727) (29.7563, 29.9922) (30.0396, 30.1636) (30.1764, 30.2463) knots 0 0 0 0 0.050568 0.097792 0.097792 0.097792 0.097792
  spline S29 degree 3 poles (30.1764, 30.2463) (30.2998, 30.3628) (30.5699, 30.6178) (30.7074, 30.964) (30.7821, 31.1522) knots 0 0 0 0 0.050293 0.110147 0.110147 0.110147 0.110147
  line L93 (27.557, 32.7402) -> (30.793, 32.7402)
  spline S30 degree 3 poles (30.793, 32.7402) (30.7682, 32.9595) (30.7236, 33.3534) (30.5146, 33.6885) (30.422, 33.837) knots 0 0 0 0 0.065203 0.117085 0.117085 0.117085 0.117085
  spline S31 degree 3 poles (30.422, 33.837) (30.2534, 34.0026) (29.9148, 34.3351) (29.4423, 34.3813) (29.205, 34.4046) knots 0 0 0 0 0.068671 0.137943 0.137943 0.137943 0.137943
  spline S32 degree 3 poles (29.205, 34.4046) (28.9895, 34.3867) (28.5638, 34.3514) (28.2314, 34.0837) (28.0673, 33.9516) knots 0 0 0 0 0.063299 0.124994 0.124994 0.124994 0.124994
  spline S33 degree 3 poles (28.0673, 33.9516) (27.9305, 33.7827) (27.644, 33.4291) (27.5869, 32.9765) (27.557, 32.7402) knots 0 0 0 0 0.063909 0.133798 0.133798 0.133798 0.133798
  line L94 (33.0304, 27.0649) -> (33.0304, 35.0812)
  line L95 (33.0304, 35.0812) -> (33.9254, 35.0812)
  line L96 (33.9254, 35.0812) -> (33.9254, 34.3282)
  spline S34 degree 3 poles (33.9254, 34.3282) (34.031, 34.4644) (34.2329, 34.725) (34.5087, 34.9052) (34.6402, 34.9912) knots 0 0 0 0 0.051297 0.098108 0.098108 0.098108 0.098108
  spline S35 degree 3 poles (34.6402, 34.9912) (34.785, 35.0556) (35.092, 35.1923) (35.4283, 35.2053) (35.6061, 35.2122) knots 0 0 0 0 0.04708 0.099893 0.099893 0.099893 0.099893
  spline S36 degree 3 poles (35.6061, 35.2122) (35.8441, 35.1977) (36.3099, 35.1694) (36.7168, 34.9416) (36.9158, 34.8302) knots 0 0 0 0 0.0705 0.138 0.138 0.138 0.138
  spline S37 degree 3 poles (36.9158, 34.8302) (37.0946, 34.687) (37.4615, 34.3929) (37.6671, 33.9696) (37.7726, 33.7525) knots 0 0 0 0 0.06782 0.139223 0.139223 0.139223 0.139223
  spline S38 degree 3 poles (37.7726, 33.7525) (37.8569, 33.5117) (38.0299, 33.018) (38.051, 32.4951) (38.0618, 32.2272) knots 0 0 0 0 0.076077 0.15601 0.15601 0.15601 0.15601
  spline S39 degree 3 poles (38.0618, 32.2272) (38.0504, 31.9424) (38.0283, 31.3914) (37.8356, 30.875) (37.7426, 30.6256) knots 0 0 0 0 0.084892 0.164238 0.164238 0.164238 0.164238
  spline S40 degree 3 poles (37.7426, 30.6256) (37.6265, 30.4036) (37.3995, 29.9694) (37.0068, 29.677) (36.8149, 29.5342) knots 0 0 0 0 0.074084 0.14489 0.14489 0.14489 0.14489
  spline S41 degree 3 poles (36.8149, 29.5342) (36.6115, 29.4236) (36.2116, 29.2062) (35.758, 29.1718) (35.5352, 29.1549) knots 0 0 0 0 0.068591 0.134825 0.134825 0.134825 0.134825
  spline S42 degree 3 poles (35.5352, 29.1549) (35.3776, 29.1626) (35.0709, 29.1774) (34.7903, 29.3018) (34.6539, 29.3623) knots 0 0 0 0 0.046877 0.091234 0.091234 0.091234 0.091234
  spline S43 degree 3 poles (34.6539, 29.3623) (34.5306, 29.4347) (34.2897, 29.5762) (34.1036, 29.7844) (34.0127, 29.8862) knots 0 0 0 0 0.042587 0.083249 0.083249 0.083249 0.083249
  line L97 (34.0127, 29.8862) -> (34.0127, 27.0649)
  line L98 (34.0127, 27.0649) -> (33.0304, 27.0649)
  spline S44 degree 3 poles (33.9199, 32.1508) (33.9273, 31.8175) (33.9403, 31.2253) (34.2413, 30.7188) (34.3729, 30.4973) knots 0 0 0 0 0.097928 0.17401 0.17401 0.17401 0.17401
  spline S45 degree 3 poles (34.3729, 30.4973) (34.5291, 30.3414) (34.834, 30.0369) (35.2613, 29.9869) (35.4697, 29.9626) knots 0 0 0 0 0.064153 0.125252 0.125252 0.125252 0.125252
  spline S46 degree 3 poles (35.4697, 29.9626) (35.6823, 29.9882) (36.1201, 30.041) (36.4311, 30.3549) (36.5911, 30.5164) knots 0 0 0 0 0.062335 0.128395 0.128395 0.128395 0.128395
  spline S47 degree 3 poles (36.5911, 30.5164) (36.7267, 30.7462) (37.0371, 31.2725) (37.0503, 31.8866) (37.0577, 32.2327) knots 0 0 0 0 0.078797 0.180491 0.180491 0.180491 0.180491
  spline S48 degree 3 poles (37.0577, 32.2327) (37.0494, 32.5644) (37.0346, 33.158) (36.7345, 33.667) (36.602, 33.8916) knots 0 0 0 0 0.09753 0.174557 0.174557 0.174557 0.174557
  spline S49 degree 3 poles (36.602, 33.8916) (36.4467, 34.0523) (36.1467, 34.3628) (35.7195, 34.4167) (35.5134, 34.4428) knots 0 0 0 0 0.064875 0.125334 0.125334 0.125334 0.125334
  spline S50 degree 3 poles (35.5134, 34.4428) (35.3063, 34.4134) (34.8679, 34.3511) (34.5635, 34.0271) (34.4029, 33.8561) knots 0 0 0 0 0.060932 0.128979 0.128979 0.128979 0.128979
  spline S51 degree 3 poles (34.4029, 33.8561) (34.2624, 33.6222) (33.9488, 33.1) (33.9302, 32.4885) (33.9199, 32.1508) knots 0 0 0 0 0.080566 0.17987 0.17987 0.17987 0.17987
  line L99 (18.5256, 16.8002) -> (18.5256, 24.8002)
  line L100 (18.5256, 24.8002) -> (20.1191, 24.8002)
  line L101 (20.1191, 24.8002) -> (22.0127, 19.1358)
  spline S52 degree 3 poles (22.0127, 19.1358) (22.0889, 18.9055) (22.2192, 18.5117) (22.3432, 18.1159) (22.3947, 17.9516) knots 0 0 0 0 0.072781 0.124428 0.124428 0.124428 0.124428
  spline S53 degree 3 poles (22.3947, 17.9516) (22.4524, 18.1314) (22.5902, 18.5603) (22.7358, 18.9865) (22.8203, 19.234) knots 0 0 0 0 0.056647 0.135122 0.135122 0.135122 0.135122
  line L102 (22.8203, 19.234) -> (24.7357, 24.8002)
  line L103 (24.7357, 24.8002) -> (26.16, 24.8002)
  line L104 (26.16, 24.8002) -> (26.16, 16.8002)
  line L105 (26.16, 16.8002) -> (25.1396, 16.8002)
  line L106 (25.1396, 16.8002) -> (25.1396, 23.496)
  line L107 (25.1396, 23.496) -> (22.8149, 16.8002)
  line L108 (22.8149, 16.8002) -> (21.8599, 16.8002)
  line L109 (21.8599, 16.8002) -> (19.5461, 23.6106)
  line L110 (19.5461, 23.6106) -> (19.5461, 16.8002)
  line L111 (19.5461, 16.8002) -> (18.5256, 16.8002)
  line L112 (31.7098, 18.6665) -> (32.7248, 18.541)
  spline S54 degree 3 poles (32.7248, 18.541) (32.6316, 18.2641) (32.4511, 17.7282) (32.036, 17.3454) (31.8353, 17.1604) knots 0 0 0 0 0.086094 0.166606 0.166606 0.166606 0.166606
  spline S55 degree 3 poles (31.8353, 17.1604) (31.5951, 17.0173) (31.0851, 16.7134) (30.4908, 16.6845) (30.1764, 16.6692) knots 0 0 0 0 0.08261 0.175377 0.175377 0.175377 0.175377
  spline S56 degree 3 poles (30.1764, 16.6692) (29.7808, 16.6955) (29.0244, 16.7456) (28.4392, 17.2241) (28.16, 17.4523) knots 0 0 0 0 0.115653 0.221163 0.221163 0.221163 0.221163
  spline S57 degree 3 poles (28.16, 17.4523) (27.9431, 17.755) (27.4744, 18.4088) (27.4359, 19.2155) (27.4151, 19.6488) knots 0 0 0 0 0.109404 0.236358 0.236358 0.236358 0.236358
  spline S58 degree 3 poles (27.4151, 19.6488) (27.4356, 20.0964) (27.4735, 20.9274) (27.9489, 21.6059) (28.1682, 21.9189) knots 0 0 0 0 0.131235 0.243597 0.243597 0.243597 0.243597
  spline S59 degree 3 poles (28.1682, 21.9189) (28.4424, 22.1544) (29.0042, 22.6369) (29.7434, 22.6962) (30.1218, 22.7265) knots 0 0 0 0 0.105595 0.216319 0.216319 0.216319 0.216319
  spline S60 degree 3 poles (30.1218, 22.7265) (30.4889, 22.6964) (31.2082, 22.6372) (31.7537, 22.166) (32.0209, 21.9353) knots 0 0 0 0 0.10743 0.210533 0.210533 0.210533 0.210533
  spline S61 degree 3 poles (32.0209, 21.9353) (32.2354, 21.6284) (32.7008, 20.9627) (32.7377, 20.148) (32.7576, 19.7088) knots 0 0 0 0 0.110094 0.23884 0.23884 0.23884 0.23884
  spline S62 degree 3 poles (32.7576, 19.7088) (32.7572, 19.6724) (32.7564, 19.5851) (32.7537, 19.4978) (32.7521, 19.4469) knots 0 0 0 0 0.010915 0.0262 0.0262 0.0262 0.0262
  line L113 (32.7521, 19.4469) -> (28.4302, 19.4469)
  spline S63 degree 3 poles (28.4302, 19.4469) (28.4585, 19.1559) (28.5109, 18.619) (28.8261, 18.1837) (28.9704, 17.9844) knots 0 0 0 0 0.08586 0.158415 0.158415 0.158415 0.158415
  spline S64 degree 3 poles (28.9704, 17.9844) (29.1434, 17.8364) (29.4926, 17.5376) (29.9507, 17.4972) (30.1819, 17.4769) knots 0 0 0 0 0.066533 0.134307 0.134307 0.134307 0.134307
  spline S65 degree 3 poles (30.1819, 17.4769) (30.353, 17.487) (30.684, 17.5066) (30.9673, 17.6779) (31.1041, 17.7606) knots 0 0 0 0 0.050568 0.097792 0.097792 0.097792 0.097792
  spline S66 degree 3 poles (31.1041, 17.7606) (31.2275, 17.8771) (31.4976, 18.1321) (31.6351, 18.4784) (31.7098, 18.6665) knots 0 0 0 0 0.050293 0.110147 0.110147 0.110147 0.110147
  line L114 (28.4847, 20.2545) -> (31.7207, 20.2545)
  spline S67 degree 3 poles (31.7207, 20.2545) (31.6959, 20.4739) (31.6513, 20.8678) (31.4423, 21.2029) (31.3497, 21.3514) knots 0 0 0 0 0.065203 0.117085 0.117085 0.117085 0.117085
  spline S68 degree 3 poles (31.3497, 21.3514) (31.1811, 21.5169) (30.8425, 21.8494) (30.37, 21.8957) (30.1327, 21.9189) knots 0 0 0 0 0.068671 0.137943 0.137943 0.137943 0.137943
  spline S69 degree 3 poles (30.1327, 21.9189) (29.9172, 21.901) (29.4915, 21.8657) (29.1591, 21.5981) (28.995, 21.466) knots 0 0 0 0 0.0633 0.124994 0.124994 0.124994 0.124994
  spline S70 degree 3 poles (28.995, 21.466) (28.8581, 21.297) (28.5717, 20.9434) (28.5146, 20.4909) (28.4847, 20.2545) knots 0 0 0 0 0.063909 0.133798 0.133798 0.133798 0.133798
  line L115 (10.5065, 4.3145) -> (10.5065, 12.3145)
  line L116 (10.5065, 12.3145) -> (16.291, 12.3145)
  line L117 (16.291, 12.3145) -> (16.291, 11.3705)
  line L118 (16.291, 11.3705) -> (11.5652, 11.3705)
  line L119 (11.5652, 11.3705) -> (11.5652, 8.9203)
  line L120 (11.5652, 8.9203) -> (15.9909, 8.9203)
  line L121 (15.9909, 8.9203) -> (15.9909, 7.9817)
  line L122 (15.9909, 7.9817) -> (11.5652, 7.9817)
  line L123 (11.5652, 7.9817) -> (11.5652, 5.2586)
  line L124 (11.5652, 5.2586) -> (16.4765, 5.2586)
  line L125 (16.4765, 5.2586) -> (16.4765, 4.3145)
  line L126 (16.4765, 4.3145) -> (10.5065, 4.3145)
  line L127 (17.8135, 4.3145) -> (17.8135, 10.1099)
  line L128 (17.8135, 10.1099) -> (18.6921, 10.1099)
  line L129 (18.6921, 10.1099) -> (18.6921, 9.2968)
  spline S71 degree 3 poles (18.6921, 9.2968) (18.7912, 9.4321) (18.9909, 9.7049) (19.2748, 9.8889) (19.4179, 9.9817) knots 0 0 0 0 0.049853 0.100536 0.100536 0.100536 0.100536
  spline S72 degree 3 poles (19.4179, 9.9817) (19.5766, 10.0572) (19.9028, 10.2126) (20.2638, 10.2313) (20.4493, 10.2409) knots 0 0 0 0 0.052187 0.107276 0.107276 0.107276 0.107276
  spline S73 degree 3 poles (20.4493, 10.2409) (20.6485, 10.2333) (21.0203, 10.2191) (21.3514, 10.0514) (21.5052, 9.9735) knots 0 0 0 0 0.058975 0.110073 0.110073 0.110073 0.110073
  spline S74 degree 3 poles (21.5052, 9.9735) (21.6327, 9.8747) (21.8901, 9.6752) (22.0205, 9.3766) (22.0864, 9.2259) knots 0 0 0 0 0.04756 0.096056 0.096056 0.096056 0.096056
  spline S75 degree 3 poles (22.0864, 9.2259) (22.3266, 9.5218) (22.7924, 10.0955) (23.5227, 10.1934) (23.8763, 10.2409) knots 0 0 0 0 0.1098 0.212838 0.212838 0.212838 0.212838
  spline S76 degree 3 poles (23.8763, 10.2409) (24.1404, 10.2274) (24.633, 10.2023) (25.0219, 9.9024) (25.2023, 9.7634) knots 0 0 0 0 0.07719 0.143952 0.143952 0.143952 0.143952
  spline S77 degree 3 poles (25.2023, 9.7634) (25.3372, 9.5677) (25.6403, 9.1278) (25.6569, 8.5908) (25.6662, 8.2927) knots 0 0 0 0 0.069911 0.157111 0.157111 0.157111 0.157111
  line L130 (25.6662, 8.2927) -> (25.6662, 4.3145)
  line L131 (25.6662, 4.3145) -> (24.6894, 4.3145)
  line L132 (24.6894, 4.3145) -> (24.6894, 7.9653)
  spline S78 degree 3 poles (24.6894, 7.9653) (24.6893, 8.1352) (24.6893, 8.4221) (24.6215, 8.7004) (24.5939, 8.8139) knots 0 0 0 0 0.050739 0.085655 0.085655 0.085655 0.085655
  spline S79 degree 3 poles (24.5939, 8.8139) (24.5548, 8.8965) (24.475, 9.0652) (24.3242, 9.1752) (24.2473, 9.2313) knots 0 0 0 0 0.026981 0.05503 0.05503 0.05503 0.05503
  spline S80 degree 3 poles (24.2473, 9.2313) (24.1582, 9.2775) (23.9735, 9.3731) (23.7656, 9.3839) (23.658, 9.3896) knots 0 0 0 0 0.029755 0.061652 0.061652 0.061652 0.061652
  spline S81 degree 3 poles (23.658, 9.3896) (23.4642, 9.3739) (23.0834, 9.3431) (22.788, 9.1016) (22.643, 8.983) knots 0 0 0 0 0.05685 0.111677 0.111677 0.111677 0.111677
  spline S82 degree 3 poles (22.643, 8.983) (22.5256, 8.8123) (22.2582, 8.4233) (22.246, 7.9482) (22.2392, 7.6815) knots 0 0 0 0 0.060926 0.138868 0.138868 0.138868 0.138868
  line L133 (22.2392, 7.6815) -> (22.2392, 4.3145)
  line L134 (22.2392, 4.3145) -> (21.2569, 4.3145)
  line L135 (21.2569, 4.3145) -> (21.2569, 8.0799)
  spline S83 degree 3 poles (21.2569, 8.0799) (21.253, 8.2752) (21.2462, 8.622) (21.0865, 8.9283) (21.0168, 9.0621) knots 0 0 0 0 0.057612 0.102327 0.102327 0.102327 0.102327
  spline S84 degree 3 poles (21.0168, 9.0621) (20.9172, 9.1575) (20.6993, 9.3661) (20.3958, 9.3813) (20.231, 9.3896) knots 0 0 0 0 0.04006 0.087699 0.087699 0.087699 0.087699
  spline S85 degree 3 poles (20.231, 9.3896) (20.0954, 9.3805) (19.8242, 9.3623) (19.5842, 9.235) (19.4643, 9.1713) knots 0 0 0 0 0.040276 0.080523 0.080523 0.080523 0.080523
  spline S86 degree 3 poles (19.4643, 9.1713) (19.3545, 9.0886) (19.1299, 8.9196) (19.0135, 8.6636) (18.954, 8.5328) knots 0 0 0 0 0.040543 0.082899 0.082899 0.082899 0.082899
  spline S87 degree 3 poles (18.954, 8.5328) (18.9081, 8.3627) (18.8011, 7.9667) (18.7977, 7.5558) (18.7958, 7.3214) knots 0 0 0 0 0.052651 0.122613 0.122613 0.122613 0.122613
  line L136 (18.7958, 7.3214) -> (18.7958, 4.3145)
  line L137 (18.7958, 4.3145) -> (17.8135, 4.3145)
  line L138 (27.1232, 2.0935) -> (27.1232, 10.1099)
  line L139 (27.1232, 10.1099) -> (28.0181, 10.1099)
  line L140 (28.0181, 10.1099) -> (28.0181, 9.3568)
  spline S88 degree 3 poles (28.0181, 9.3568) (28.1237, 9.4931) (28.3257, 9.7536) (28.6015, 9.9339) (28.733, 10.0199) knots 0 0 0 0 0.051297 0.098108 0.098108 0.098108 0.098108
  spline S89 degree 3 poles (28.733, 10.0199) (28.8777, 10.0843) (29.1848, 10.2209) (29.5211, 10.234) (29.6989, 10.2409) knots 0 0 0 0 0.04708 0.099894 0.099894 0.099894 0.099894
  spline S90 degree 3 poles (29.6989, 10.2409) (29.9369, 10.2264) (30.4026, 10.198) (30.8096, 9.9703) (31.0086, 9.8589) knots 0 0 0 0 0.0705 0.138 0.138 0.138 0.138
  spline S91 degree 3 poles (31.0086, 9.8589) (31.1873, 9.7156) (31.5543, 9.4215) (31.7599, 8.9982) (31.8653, 8.7811) knots 0 0 0 0 0.06782 0.139223 0.139223 0.139223 0.139223
  spline S92 degree 3 poles (31.8653, 8.7811) (31.9497, 8.5404) (32.1226, 8.0467) (32.1438, 7.5238) (32.1546, 7.2559) knots 0 0 0 0 0.076078 0.156009 0.156009 0.156009 0.156009
  spline S93 degree 3 poles (32.1546, 7.2559) (32.1432, 6.9711) (32.1211, 6.4201) (31.9284, 5.9037) (31.8353, 5.6542) knots 0 0 0 0 0.084892 0.164238 0.164238 0.164238 0.164238
  spline S94 degree 3 poles (31.8353, 5.6542) (31.7193, 5.4322) (31.4922, 4.9981) (31.0995, 4.7057) (30.9076, 4.5628) knots 0 0 0 0 0.074084 0.144891 0.144891 0.144891 0.144891
  spline S95 degree 3 poles (30.9076, 4.5628) (30.7042, 4.4522) (30.3044, 4.2348) (29.8508, 4.2004) (29.628, 4.1836) knots 0 0 0 0 0.068591 0.134825 0.134825 0.134825 0.134825
  spline S96 degree 3 poles (29.628, 4.1836) (29.4704, 4.1912) (29.1636, 4.2061) (28.8831, 4.3305) (28.7467, 4.3909) knots 0 0 0 0 0.046877 0.091235 0.091235 0.091235 0.091235
  spline S97 degree 3 poles (28.7467, 4.3909) (28.6234, 4.4633) (28.3825, 4.6049) (28.1964, 4.8131) (28.1055, 4.9148) knots 0 0 0 0 0.042587 0.083249 0.083249 0.083249 0.083249
  line L141 (28.1055, 4.9148) -> (28.1055, 2.0935)
  line L142 (28.1055, 2.0935) -> (27.1232, 2.0935)
  spline S98 degree 3 poles (28.0127, 7.1795) (28.02, 6.8462) (28.0331, 6.254) (28.334, 5.7475) (28.4656, 5.526) knots 0 0 0 0 0.097928 0.174009 0.174009 0.174009 0.174009
  spline S99 degree 3 poles (28.4656, 5.526) (28.6218, 5.37) (28.9268, 5.0656) (29.3541, 5.0156) (29.5625, 4.9912) knots 0 0 0 0 0.064153 0.125251 0.125251 0.125251 0.125251